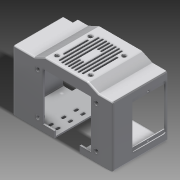
# Autodesk Inventor part: Simple3DPrintEnclosure02
Saved by Autodesk Inventor 2015 (Build 190159000, 159)
## iProperties
Created: 2015-09-24
Part Number: Simple3DPrintEnclosure02
Material: Aluminum 6061 Black Anodized
Document SubType Name: Modeling
Designer: -
Density: 2.71 g/cm^3
Appearance: Aluminum - Polished
Mass: 237.828 g
Surface Area: 585.089 cm^2
Volume: 87.7595 cm^3
Author: -
Autodesk Inventor part; units mm, degrees
ref_plane "YZ Plane" through (0, 0, 0) normal (1, 0, 0) x (0, 1, 0)
ref_plane "XZ Plane" through (0, 0, 0) normal (0, 1, 0) x (-1, 0, 0)
ref_plane "XY Plane" through (0, 0, 0) normal (0, 0, 1) x (1, 0, 0)
ref_plane "Work Plane1" through (-36.1295, 16.7619, 114.6398) normal (0, 0, 1) x (1, 0, 0)
sketch "Sketch3" plane through (-36.1295, 16.7619, 114.6398) normal (0, 0, 1) x (1, 0, 0)
  line L0 (55.17, 45.25) -> (-64.79, 45.25)
  line L1 (-64.79, 45.25) -> (-64.79, -34.1)
  line L2 (-64.79, -34.1) -> (55.17, -34.1)
  line L3 (55.17, -34.1) -> (55.17, 45.25)
  line L4 (28.95, 31.25) -> (28.95, -26.1)
  line L5 (-28.4, 31.25) -> (28.95, 31.25)
  line L6 (-28.4, -26.1) -> (-28.4, 31.25)
  line L7 (28.95, -26.1) -> (-28.4, -26.1)
  line L8 (28.95, 31.25) -> (-28.4, 31.25)
  line L9 (-28.4, 31.25) -> (-28.4, -26.1)
  line L10 (-28.4, -26.1) -> (28.95, -26.1)
  line L11 (28.95, -26.1) -> (28.95, 31.25)
  dimension "d196" = 14
  dimension "d197" = 26.22
  dimension "d198" = 8
  dimension "d199" = 36.39
  dimension "d200" = 57.35
  dimension "d201" = 57.35
  dimension "d249" = 119.96
  constraints: 24 end point, 4 parallel, 2 horizontal, 2 perpendicular
  measures "d196" distance between parallel lines of L0 L5
  measures "d197" distance between parallel lines of L3 L4
  measures "d198" distance between parallel lines of L2 L7
  measures "d199" distance between parallel lines of L1 L6
  measures "d200" distance between parallel lines of L5 L10
  measures "d201" distance between parallel lines of L6 L11
  measures "d249" distance between parallel lines of L3 L1
extrude "Extrusion3" add sketch "Sketch3" along normal blind 2
sketch "Sketch4" plane through (-36.1295, 16.7619, 114.6398) normal (0, 0, -1) x (-1, 0, 0)
  line L0 (-55.17, 45.25) -> (64.79, 45.25) projected
  line L1 (-55.17, -34.1) -> (-55.17, 45.25) projected
  line L2 (64.79, -34.1) -> (-55.17, -34.1) projected
  line L3 (64.79, 45.25) -> (64.79, -34.1) projected
  line L4 (-53.17, -32.1) -> (62.79, -32.1)
  line L5 (-23.5099, 42.25) -> (25.1599, 42.25)
  line L6 (64.79, -34.1) -> (-55.17, -34.1) construction
  line L7 (4.81, -34.1) -> (4.81, -47.8213) construction
  line L8 (29.4, 28.05) -> (-27.75, 28.05) construction
  line L9 (0.825, 28.05) -> (0.825, 13.0921) construction
  line L10 (-55.17, 45.25) -> (64.79, 45.25) projected
  line L11 (-24.7778, 41.9689) -> (-36.5722, 36.4691)
  line L12 (-37.8401, 36.188) -> (-53.17, 36.188)
  line L13 (26.4278, 41.9689) -> (38.2222, 36.4691)
  line L14 (39.4901, 36.188) -> (62.79, 36.188)
  line L15 (64.79, 45.25) -> (64.79, -34.1) projected
  arc A0 (-37.8401, 36.188) -> (-36.5722, 36.4691) centre (-37.8401, 39.188) ccw
  arc A1 (-23.5099, 42.25) -> (-24.7778, 41.9689) centre (-23.5099, 39.25) ccw
  arc A2 (26.4278, 41.9689) -> (25.1599, 42.25) centre (25.1599, 39.25) ccw
  arc A3 (38.2222, 36.4691) -> (39.4901, 36.188) centre (39.4901, 39.188) ccw
  line L16 (-55.17, 38.188) -> (-37.8401, 38.188)
  arc A4 (-37.8401, 38.188) -> (-37.4175, 38.2817) centre (-37.8401, 39.188) ccw
  line L17 (-37.4175, 38.2817) -> (-25.623, 43.7815)
  arc A5 (-23.5099, 44.25) -> (-25.623, 43.7815) centre (-23.5099, 39.25) ccw
  line L18 (-23.5099, 44.25) -> (25.1599, 44.25)
  arc A6 (27.273, 43.7815) -> (25.1599, 44.25) centre (25.1599, 39.25) ccw
  line L19 (27.273, 43.7815) -> (39.0675, 38.2817)
  arc A7 (39.0675, 38.2817) -> (39.4901, 38.188) centre (39.4901, 39.188) ccw
  line L20 (39.4901, 38.188) -> (64.79, 38.188)
  line L21 (62.79, -32.1) -> (62.79, 36.188)
  line L22 (-53.17, -32.1) -> (-53.17, 36.188)
  line L23 (-55.17, 38.188) -> (-55.17, -34.1)
  line L24 (64.79, -34.1) -> (64.79, 38.188)
  point P0 (-36.1295, -16.7619)
  point P1 (-24.175, 42.25)
  point P2 (25.825, 42.25)
  point P3 (-37.175, 36.188)
  point P4 (38.825, 36.188)
  point P5 (0.825, 42.25)
  dimension "d70" = 3
  dimension "d71" = 155
  dimension "d72" = 13
  dimension "d73" = 50
  dimension "d74" = 155
  dimension "d75" = 13
  dimension "d76" = 3
  dimension "d77" = 2
  dimension "d78" = 2
  dimension "d79" = 2
  dimension "d204" = 2
  dimension "d205" = 2
  dimension "d206" = 2
  dimension "d250" = 115.96
  dimension "d263" = 39.6301
  dimension "d264" = 31.6601
  dimension "d265" = 72.288
  constraints: 34 end point, 16 point on circle, 9 point on line, 8 centre point, 8 tangent, 3 equal radius, 3 horizontal, 3 midpoint, 2 collinear, 2 perpendicular, 2 vertical, 6 other
  measures "d70" distance between parallel lines of L5 L0
  measures "d71" angle of L11 L5
  measures "d72" horizontal distance of point (-37.175, 36.188) point (-24.175, 42.25)
  measures "d73" distance of point (-24.175, 42.25) point (25.825, 42.25)
  measures "d74" angle of L13 L5
  measures "d75" horizontal distance of point (25.825, 42.25) point (38.825, 36.188)
  measures "d76" radius of A0
  measures "d77" distance between parallel lines of L11 L17
  measures "d78" distance between parallel lines of L20 L14
  measures "d79" distance between parallel lines of L16 L12
  measures "d204" distance between parallel lines of L2 L4
  measures "d205" distance between parallel lines of L1 L22
  measures "d206" distance between parallel lines of L3 L21
  measures "d250" distance between parallel lines of L21 L22
  measures "d263" distance from line of L18.end L3
  measures "d264" distance from line of L1 L18.start
  measures "d265" distance between parallel lines of L2 L16
extrude "Extrusion4" add sketch "Sketch4" along normal blind 63 contours L16 A4 L17 A5 L18 A6 L19 A7 L20 L3 L2 L1
sketch "Sketch9" plane through (-36.1295, 16.7619, 114.6398) normal (0, 0, -1) x (-1, 0, 0)
  arc A0 (-23.5099, 44.25) -> (-25.623, 43.7815) centre (-23.5099, 39.25) ccw projected
  line L0 (-55.17, 45.25) -> (64.79, 45.25) projected
  line L1 (-55.17, 38.188) -> (-55.17, 45.25) projected
  line L2 (-55.17, 38.188) -> (-37.8401, 38.188) projected
  line L3 (-37.4175, 38.2817) -> (-25.623, 43.7815) projected
  arc A1 (27.273, 43.7815) -> (25.1599, 44.25) centre (25.1599, 39.25) ccw projected
  line L4 (27.273, 43.7815) -> (39.0675, 38.2817) projected
  line L5 (39.4901, 38.188) -> (64.79, 38.188) projected
  line L6 (64.79, 45.25) -> (64.79, 38.188) projected
  line L7 (-55.17, 45.25) -> (64.79, 45.25) projected
  line L8 (-55.17, 38.188) -> (-55.17, 45.25) projected
  line L9 (-55.17, 38.188) -> (-37.8401, 38.188) projected
  line L10 (-37.4175, 38.2817) -> (-25.623, 43.7815) projected
  arc A2 (-23.5099, 44.25) -> (-25.623, 43.7815) centre (-23.5099, 39.25) ccw projected
  line L11 (39.4901, 38.188) -> (64.79, 38.188) projected
  line L12 (64.79, 45.25) -> (64.79, 38.188) projected
  arc A3 (27.273, 43.7815) -> (25.1599, 44.25) centre (25.1599, 39.25) ccw projected
  line L13 (27.273, 43.7815) -> (39.0675, 38.2817) projected
  arc A4 (-37.8401, 38.188) -> (-37.4175, 38.2817) centre (-37.8401, 39.188) ccw projected
  line L14 (-23.5099, 44.25) -> (25.1599, 44.25) projected
  arc A5 (39.0675, 38.2817) -> (39.4901, 38.188) centre (39.4901, 39.188) ccw projected
  arc A6 (-37.8401, 38.188) -> (-37.4175, 38.2817) centre (-37.8401, 39.188) ccw projected
  line L15 (-23.5099, 44.25) -> (25.1599, 44.25) projected
  arc A7 (39.0675, 38.2817) -> (39.4901, 38.188) centre (39.4901, 39.188) ccw projected
  point P0 (-36.1295, -16.7619)
extrude "Extrusion9" cut sketch "Sketch9" against normal blind 6
fillet "Fillet16" radius 2 12 edges at (-100.9195, 54.9499, 84.1398) (19.0405, 54.9499, 84.1398) (19.0405, -17.3381, 84.1398) (-100.9195, -17.3381, 84.1398) (-88.2695, 54.9499, 116.6398) (-100.9195, 18.8059, 116.6398) (19.0405, 18.8059, 116.6398) (10.3756, 54.9499, 116.6398) (-11.5374, 60.8934, 116.6398) (-62.3716, 60.8934, 116.6398) (-69.2997, 57.7936, 116.6398) (-4.6093, 57.7936, 116.6398)
chamfer "Chamfer1" [suppressed]
chamfer "Chamfer2" [suppressed]
chamfer "Chamfer5" [suppressed]
fillet "Fillet5" [suppressed]
fillet "Fillet6" [suppressed]
fillet "Fillet14" [suppressed]
sketch "Sketch7" plane through (19.0405, -15.3381, 51.6398) normal (1, 0, 0) x (0, 0, -1)
  line L0 (-40, 62) -> (-4, 62)
  line L1 (-2, 60) -> (-2, 9)
  line L2 (-4, 7) -> (-40, 7)
  line L3 (-42, 9) -> (-42, 60)
  arc A0 (-40, 62) -> (-42, 60) centre (-40, 60) ccw
  arc A1 (-2, 60) -> (-4, 62) centre (-4, 60) ccw
  arc A2 (-4, 7) -> (-2, 9) centre (-4, 9) ccw
  arc A3 (-42, 9) -> (-40, 7) centre (-40, 9) ccw
  line L4 (0, 68.288) -> (0, 0) projected
  line L5 (-64, -2) -> (0, -2) projected
  point P0 (51.6398, 15.3381)
  point P1 (0, 69.288)
  point P2 (-64.7639, -2)
  point P3 (-63.5279, -2)
  dimension "d46" = 2
  dimension "d65" = 40
  dimension "d66" = 55
  dimension "d240" = 2
  dimension "d241" = 9
  constraints: 8 end point, 8 point on circle, 8 tangent, 4 centre point, 3 equal radius, 2 parallel, 1 horizontal, 1 perpendicular
  measures "d46" radius of A0
  measures "d65" distance between parallel lines of L3 L1
  measures "d66" distance between parallel lines of L2 L0
  measures "d240" distance between parallel lines of L1 L4
  measures "d241" distance between parallel lines of L5 L2
extrude "Extrusion7" cut sketch "Sketch7" against normal blind 1
lip "Lip1" kind groove height 1 width 1 edges at (-40.9395, -15.3381, 51.6398) (-98.9195, 18.8059, 51.6398) (-87.2695, 52.9499, 51.6398) (-74.9703, 53.021, 51.6398) (-68.4545, 55.9809, 51.6398) (-61.9387, 58.9408, 51.6398) (-36.9545, 59.0119, 51.6398) (-11.9703, 58.9408, 51.6398) (-5.4545, 55.9809, 51.6398) (1.0613, 53.021, 51.6398) (9.3756, 52.9499, 51.6398) (17.0405, 18.8059, 51.6398) guide face at (-60.2662, -16.0047, 51.6398)
sketch "Sketch16" plane through (18.0405, -15.3381, 51.6398) normal (1, 0, 0) x (0, 0, -1)
  line L0 (-2, 60) -> (-2, 9) projected
  line L1 (-42, 58) -> (-2, 58)
  line L2 (-2, 58) -> (-2, 11)
  line L3 (-2, 11) -> (-42, 11)
  line L4 (-42, 11) -> (-42, 58)
  line L5 (-40, 62) -> (-4, 62) projected
  line L6 (-4, 7) -> (-40, 7) projected
  line L7 (-42, 9) -> (-42, 60) projected
  circle A0 centre (-22, 9) radius 1
  line L8 (-22, 11) -> (-22, 7) construction
  line L9 (-4, 7) -> (-40, 7) construction
  circle A1 centre (-22, 60) radius 1
  line L10 (-22, 58) -> (-22, 62) construction
  point P0 (51.6398, 15.3381)
  dimension "d243" = 4
  dimension "d244" = 4
  dimension "d247" = 2
  dimension "d248" = 2
  constraints: 12 end point, 7 midpoint, 2 centre point, 2 coincident, 2 parallel, 1 collinear, 1 horizontal, 1 perpendicular, 1 point on line
  measures "d243" distance between parallel lines of L5 L1
  measures "d244" distance between parallel lines of L6 L3
  measures "d247" diameter of A0
  measures "d248" diameter of A1
extrude "Extrusion15" cut sketch "Sketch16" against normal blind 10
sketch "Sketch8" plane through (-36.1295, 16.7619, 116.6398) normal (0, 0, 1) x (1, 0, 0)
  circle A0 centre (-34.95, 27.44) radius 1.5
  circle A1 centre (-34.95, -22.29) radius 1.5
  line L0 (0, 0) -> (0, 75.8555) construction
  circle A2 centre (34.95, 27.44) radius 1.5
  circle A3 centre (34.95, -22.29) radius 1.5
  line L1 (0, 0) -> (67.5955, 0) construction
  line L2 (-28.4, 31.25) -> (28.95, 31.25) projected
  line L3 (28.95, 31.25) -> (28.95, -26.1) projected
  line L4 (28.95, -26.1) -> (-28.4, -26.1) projected
  point P0 (0, 28.05)
  dimension "d55" = 3
  dimension "d58" = 3
  dimension "d259" = 3.81
  dimension "d260" = 6
  dimension "d261" = 6
  dimension "d262" = 3.81
  constraints: 4 centre point, 4 end point, 2 point on line, 2 symmetric about line, 1 horizontal, 1 vertical, 3 other
  measures "d55" diameter of A0
  measures "d58" diameter of A1
  measures "d259" distance from line of A2.centre L2
  measures "d260" distance from line of A2.centre L3
  measures "d261" distance from line of L3 A3.centre
  measures "d262" distance from line of L4 A3.centre
extrude "Extrusion8" cut sketch "Sketch8" against normal blind 6
chamfer "Chamfer4" distance 1.2 angle 45 4 edges at (-72.5795, 44.2019, 116.6398) (-72.5795, -5.5281, 116.6398) (-2.6795, 44.2019, 116.6398) (-2.6795, -5.5281, 116.6398)
fillet "Fillet11" radius 1 4 edges at (-3.8795, -5.5281, 116.6398) (-3.8795, 44.2019, 116.6398) (-73.7795, 44.2019, 116.6398) (-73.7795, -5.5281, 116.6398)
fillet "Fillet12" radius 2 8 edges at (-98.9195, -15.3381, 83.6398) (-99.9195, -16.3381, 52.1398) (17.0405, -15.3381, 83.6398) (18.0405, -16.3381, 52.1398) (17.0405, 52.9499, 83.6398) (18.0405, 53.9499, 52.1398) (-98.9195, 52.9499, 83.6398) (-99.9195, 53.9499, 52.1398)
sketch "Sketch10" plane through (-61.2894, 61.0119, 51.6398) normal (0, 1, 0) x (1, 0, 0)
  line L0 (49.1988, -64.7639) -> (-0.8012, -64.7639) construction
  line L1 (-0.8012, -64.7639) -> (-0.8012, -14.7639) construction
  line L2 (-0.8012, -14.7639) -> (49.1988, -14.7639) construction
  line L3 (49.1988, -14.7639) -> (49.1988, -64.7639) construction
  line L4 (48.6698, -64) -> (48.6698, 0) construction
  line L5 (0, 0) -> (48.6698, 0) construction
  line L6 (0, -64) -> (0, 0) construction
  circle A0 centre (4.1988, -15.7639) radius 1.75
  line L7 (48.6698, 0) -> (0, 0) construction
  line L8 (24.3349, 0) -> (24.3349, 10.9625) construction
  circle A1 centre (44.471, -15.7639) radius 1.75
  circle A2 centre (4.1988, -55.7639) radius 1.75
  circle A3 centre (44.471, -55.7639) radius 1.75
  line L9 (42.221, -50.7639) -> (42.221, -50.7639)
  line L10 (43.221, -49.7639) -> (43.221, -21.7639)
  line L11 (42.221, -20.7639) -> (42.221, -20.7639)
  line L12 (41.221, -21.7639) -> (41.221, -49.7639)
  line L13 (39.2176, -35.7639) -> (24.1918, -35.7639) construction
  line L14 (44.471, -55.7639) -> (44.471, -15.7639) construction
  arc A4 (41.221, -49.7639) -> (42.221, -50.7639) centre (42.221, -49.7639) ccw
  arc A5 (42.221, -50.7639) -> (43.221, -49.7639) centre (42.221, -49.7639) ccw
  arc A6 (43.221, -21.7639) -> (42.221, -20.7639) centre (42.221, -21.7639) ccw
  arc A7 (42.221, -20.7639) -> (41.221, -21.7639) centre (42.221, -21.7639) ccw
  line L15 (38.221, -59.7639) -> (38.221, -59.7639)
  line L16 (39.221, -58.7639) -> (39.221, -12.7639)
  line L17 (38.221, -11.7639) -> (38.221, -11.7639)
  line L18 (37.221, -12.7639) -> (37.221, -58.7639)
  arc A8 (37.221, -58.7639) -> (38.221, -59.7639) centre (38.221, -58.7639) ccw
  arc A9 (38.221, -59.7639) -> (39.221, -58.7639) centre (38.221, -58.7639) ccw
  arc A10 (39.221, -12.7639) -> (38.221, -11.7639) centre (38.221, -12.7639) ccw
  arc A11 (38.221, -11.7639) -> (37.221, -12.7639) centre (38.221, -12.7639) ccw
  line L19 (34.221, -60.7639) -> (34.221, -60.7639)
  line L20 (35.221, -59.7639) -> (35.221, -11.7639)
  line L21 (34.221, -10.7639) -> (34.221, -10.7639)
  line L22 (33.221, -11.7639) -> (33.221, -59.7639)
  arc A12 (33.221, -59.7639) -> (34.221, -60.7639) centre (34.221, -59.7639) ccw
  arc A13 (34.221, -60.7639) -> (35.221, -59.7639) centre (34.221, -59.7639) ccw
  arc A14 (35.221, -11.7639) -> (34.221, -10.7639) centre (34.221, -11.7639) ccw
  arc A15 (34.221, -10.7639) -> (33.221, -11.7639) centre (34.221, -11.7639) ccw
  line L23 (26.221, -10.7639) -> (26.221, -10.7639)
  line L24 (27.221, -11.7639) -> (27.221, -24.7639)
  line L25 (26.221, -25.7639) -> (26.221, -25.7639)
  line L26 (25.221, -24.7639) -> (25.221, -11.7639)
  arc A16 (26.221, -10.7639) -> (25.221, -11.7639) centre (26.221, -11.7639) ccw
  arc A17 (27.221, -11.7639) -> (26.221, -10.7639) centre (26.221, -11.7639) ccw
  arc A18 (26.221, -25.7639) -> (27.221, -24.7639) centre (26.221, -24.7639) ccw
  arc A19 (25.221, -24.7639) -> (26.221, -25.7639) centre (26.221, -24.7639) ccw
  line L27 (49.471, -14.7639) -> (-0.529, -14.7639) construction
  line L28 (22.4488, -10.7639) -> (22.4488, -10.7639)
  line L29 (21.4488, -11.7639) -> (21.4488, -24.7639)
  line L30 (22.4488, -25.7639) -> (22.4488, -25.7639)
  line L31 (23.4488, -24.7639) -> (23.4488, -11.7639)
  arc A20 (23.4488, -11.7639) -> (22.4488, -10.7639) centre (22.4488, -11.7639) ccw
  arc A21 (22.4488, -10.7639) -> (21.4488, -11.7639) centre (22.4488, -11.7639) ccw
  arc A22 (21.4488, -24.7639) -> (22.4488, -25.7639) centre (22.4488, -24.7639) ccw
  arc A23 (22.4488, -25.7639) -> (23.4488, -24.7639) centre (22.4488, -24.7639) ccw
  line L32 (30.221, -60.7639) -> (30.221, -60.7639)
  line L33 (31.221, -59.7639) -> (31.221, -11.7639)
  line L34 (30.221, -10.7639) -> (30.221, -10.7639)
  line L35 (29.221, -11.7639) -> (29.221, -59.7639)
  arc A24 (29.221, -59.7639) -> (30.221, -60.7639) centre (30.221, -59.7639) ccw
  arc A25 (30.221, -60.7639) -> (31.221, -59.7639) centre (30.221, -59.7639) ccw
  arc A26 (31.221, -11.7639) -> (30.221, -10.7639) centre (30.221, -11.7639) ccw
  arc A27 (30.221, -10.7639) -> (29.221, -11.7639) centre (30.221, -11.7639) ccw
  line L36 (26.221, -45.7639) -> (26.221, -45.7639)
  line L37 (27.221, -46.7639) -> (27.221, -59.7639)
  line L38 (26.221, -60.7639) -> (26.221, -60.7639)
  line L39 (25.221, -59.7639) -> (25.221, -46.7639)
  arc A28 (26.221, -45.7639) -> (25.221, -46.7639) centre (26.221, -46.7639) ccw
  arc A29 (27.221, -46.7639) -> (26.221, -45.7639) centre (26.221, -46.7639) ccw
  arc A30 (26.221, -60.7639) -> (27.221, -59.7639) centre (26.221, -59.7639) ccw
  arc A31 (25.221, -59.7639) -> (26.221, -60.7639) centre (26.221, -59.7639) ccw
  arc A32 (22.4488, -45.7639) -> (21.4488, -46.7639) centre (22.4488, -46.7639) ccw
  line L40 (22.4488, -45.7639) -> (22.4488, -45.7639)
  arc A33 (23.4488, -46.7639) -> (22.4488, -45.7639) centre (22.4488, -46.7639) ccw
  line L41 (21.4488, -46.7639) -> (21.4488, -59.7639)
  line L42 (23.4488, -59.7639) -> (23.4488, -46.7639)
  arc A34 (22.4488, -60.7639) -> (23.4488, -59.7639) centre (22.4488, -59.7639) ccw
  line L43 (22.4488, -60.7639) -> (22.4488, -60.7639)
  arc A35 (21.4488, -59.7639) -> (22.4488, -60.7639) centre (22.4488, -59.7639) ccw
  line L44 (18.721, -60.7639) -> (18.721, -60.7639)
  line L45 (19.721, -59.7639) -> (19.721, -11.7639)
  line L46 (18.721, -10.7639) -> (18.721, -10.7639)
  line L47 (17.721, -11.7639) -> (17.721, -59.7639)
  arc A36 (17.721, -59.7639) -> (18.721, -60.7639) centre (18.721, -59.7639) ccw
  arc A37 (18.721, -60.7639) -> (19.721, -59.7639) centre (18.721, -59.7639) ccw
  arc A38 (19.721, -11.7639) -> (18.721, -10.7639) centre (18.721, -11.7639) ccw
  arc A39 (18.721, -10.7639) -> (17.721, -11.7639) centre (18.721, -11.7639) ccw
  line L48 (14.721, -60.7639) -> (14.721, -60.7639)
  line L49 (15.721, -59.7639) -> (15.721, -11.7639)
  line L50 (14.721, -10.7639) -> (14.721, -10.7639)
  line L51 (13.721, -11.7639) -> (13.721, -59.7639)
  arc A40 (13.721, -59.7639) -> (14.721, -60.7639) centre (14.721, -59.7639) ccw
  arc A41 (14.721, -60.7639) -> (15.721, -59.7639) centre (14.721, -59.7639) ccw
  arc A42 (15.721, -11.7639) -> (14.721, -10.7639) centre (14.721, -11.7639) ccw
  arc A43 (14.721, -10.7639) -> (13.721, -11.7639) centre (14.721, -11.7639) ccw
  line L52 (10.721, -59.7639) -> (10.721, -59.7639)
  line L53 (11.721, -58.7639) -> (11.721, -12.7639)
  line L54 (10.721, -11.7639) -> (10.721, -11.7639)
  line L55 (9.721, -12.7639) -> (9.721, -58.7639)
  arc A44 (9.721, -58.7639) -> (10.721, -59.7639) centre (10.721, -58.7639) ccw
  arc A45 (10.721, -59.7639) -> (11.721, -58.7639) centre (10.721, -58.7639) ccw
  arc A46 (11.721, -12.7639) -> (10.721, -11.7639) centre (10.721, -12.7639) ccw
  arc A47 (10.721, -11.7639) -> (9.721, -12.7639) centre (10.721, -12.7639) ccw
  line L56 (6.721, -50.7639) -> (6.721, -50.7639)
  line L57 (7.721, -49.7639) -> (7.721, -21.7639)
  line L58 (6.721, -20.7639) -> (6.721, -20.7639)
  line L59 (5.721, -21.7639) -> (5.721, -49.7639)
  arc A48 (5.721, -49.7639) -> (6.721, -50.7639) centre (6.721, -49.7639) ccw
  arc A49 (6.721, -50.7639) -> (7.721, -49.7639) centre (6.721, -49.7639) ccw
  arc A50 (7.721, -21.7639) -> (6.721, -20.7639) centre (6.721, -21.7639) ccw
  arc A51 (6.721, -20.7639) -> (5.721, -21.7639) centre (6.721, -21.7639) ccw
  line L60 (48.6698, -64) -> (0, -64)
  point P0 (61.2894, 51.6398)
  point P1 (24.1988, -64.7639)
  point P2 (49.061, -66.2512)
  point P3 (41.221, -35.7639)
  point P4 (44.471, -35.7639)
  point P5 (39.221, -11.7639)
  point P6 (39.221, -59.7639)
  point P7 (37.221, -11.7639)
  point P8 (37.221, -35.7639)
  point P9 (35.221, -10.7639)
  point P10 (35.221, -60.7639)
  point P11 (33.221, -10.7639)
  point P12 (33.221, -35.7639)
  point P13 (27.221, -25.7639)
  point P14 (27.221, -10.7639)
  point P15 (25.221, -25.7639)
  point P16 (21.4488, -25.7639)
  point P17 (21.4488, -10.7639)
  point P18 (23.4488, -25.7639)
  point P19 (31.221, -10.7639)
  point P20 (31.221, -60.7639)
  point P21 (29.221, -10.7639)
  point P22 (29.221, -35.7639)
  point P23 (27.221, -60.7639)
  point P24 (27.221, -45.7639)
  point P25 (25.221, -60.7639)
  point P26 (21.4488, -45.7639)
  point P27 (23.4488, -60.7639)
  point P28 (21.4488, -60.7639)
  point P29 (19.721, -10.7639)
  point P30 (19.721, -60.7639)
  point P31 (17.721, -10.7639)
  point P32 (17.721, -35.7639)
  point P33 (15.721, -10.7639)
  point P34 (15.721, -60.7639)
  point P35 (13.721, -10.7639)
  point P36 (13.721, -35.7639)
  point P37 (11.7176, -35.7639)
  point P38 (11.721, -11.7639)
  point P39 (11.721, -59.7639)
  point P40 (9.721, -11.7639)
  point P41 (9.721, -35.7639)
  point P42 (5.721, -35.7639)
  dimension "d87" = 50
  dimension "d88" = 50
  dimension "d108" = 3.5
  dimension "d109" = 5
  dimension "d112" = 40
  dimension "d117" = 40
  dimension "d118" = 40.2722
  dimension "d119" = 9
  dimension "d121" = 30
  dimension "d123" = 2
  dimension "d124" = 1
  dimension "d125" = 2.5
  dimension "d131" = 2
  dimension "d132" = 48
  dimension "d133" = 2
  dimension "d134" = 1
  dimension "d135" = 2
  dimension "d136" = 50
  dimension "d137" = 2
  dimension "d138" = 1
  dimension "d147" = 2
  dimension "d148" = 15
  dimension "d151" = 1
  dimension "d152" = 2
  dimension "d153" = 50
  dimension "d154" = 2
  dimension "d155" = 1
  dimension "d156" = 2
  dimension "d157" = 1
  dimension "d160" = 35
  dimension "d167" = 15.5
  dimension "d172" = 9.5
  dimension "d175" = 27.5
  dimension "d180" = 2
  dimension "d183" = 35.5
  dimension "d188" = 2
  constraints: 122 end point, 96 point on circle, 65 point on line, 52 centre point, 40 tangent, 18 symmetric about line, 15 equal radius, 12 parallel, 9 horizontal, 7 midpoint, 7 perpendicular, 3 vertical, 124 other
  measures "d87" distance of L1.end L2.end
  measures "d88" distance of L0.end L1.end
  measures "d108" diameter of A0
  measures "d109" distance from line of A0.centre L1
  measures "d112" distance of A0.centre A2.centre
  measures "d117" distance of L14.start L14.end
  measures "d118" distance of L14.end A0.centre
  measures "d119" distance from line of A2.centre L0
  measures "d121" distance between parallel lines of L11 L9
  measures "d123" distance between parallel lines of L10 L12
  measures "d124" radius of A4
  measures "d125" diameter of L10 L14
  measures "d131" distance of point (37.221, -11.764) point (39.221, -11.764)
  measures "d132" distance of point (39.221, -11.764) point (39.221, -59.764)
  measures "d133" distance between parallel lines of L12 L16
  measures "d134" radius of A8
  measures "d135" distance of point (33.221, -10.764) point (35.221, -10.764)
  measures "d136" distance of point (35.221, -10.764) point (35.221, -60.764)
  measures "d137" distance between parallel lines of L20 L18
  measures "d138" radius of A12
  measures "d147" distance of point (27.221, -25.764) point (25.221, -25.764)
  measures "d148" distance of point (27.221, -10.764) point (27.221, -25.764)
  measures "d151" radius of A16
  measures "d152" distance of point (29.221, -10.764) point (31.221, -10.764)
  measures "d153" distance of point (31.221, -10.764) point (31.221, -60.764)
  measures "d154" distance between parallel lines of L22 L33
  measures "d155" radius of A24
  measures "d156" distance between parallel lines of L24 L35
  measures "d157" vertical distance of point (29.221, -10.764) A17.centre
  measures "d160" distance of L24.start L37.start
  measures "d167" distance of point (29.221, -35.764) point (13.721, -35.764)
  measures "d172" distance between parallel lines of L35 L45
  measures "d175" distance of point (37.221, -11.764) point (9.721, -11.764)
  measures "d180" distance between parallel lines of L51 L53
  measures "d183" distance of L11.start L58.start
  measures "d188" distance between parallel lines of L57 L55
extrude "Extrusion10" cut sketch "Sketch10" against normal blind 10
sketch "Sketch11" plane through (-97.9195, -17.3381, 51.6398) normal (0, -1, 0) x (1, 0, 0)
  line L0 (62.065, 68) -> (62.065, 29.2393) construction
  line L1 (46.965, 65) -> (77.165, 65)
  line L2 (77.165, 65) -> (77.165, 20.9)
  line L3 (77.165, 20.9) -> (46.965, 20.9)
  line L4 (46.965, 20.9) -> (46.965, 65)
  line L5 (90.74, 65) -> (33.39, 65) projected
  point P0 (97.9195, -51.6398)
  point P1 (62.065, 65)
  point P2 (62.065, 65)
  dimension "d104" = 30.2
  dimension "d266" = 44.1
  constraints: 10 end point, 2 midpoint, 2 parallel, 2 point on line, 1 collinear, 1 horizontal, 1 perpendicular, 1 vertical
  measures "d104" distance of L1.start L1.end
  measures "d266" distance between parallel lines of L3 L1
extrude "Extrusion11" cut sketch "Sketch11" against normal blind 10
sketch "Sketch13" plane through (-36.1295, 16.7619, 114.6398) normal (0, 0, -1) x (-1, 0, 0)
  line L0 (40.7978, -31.225) -> (64.4775, -31.225) projected
  line L1 (43.8489, 33.1934) -> (43.8489, -32.2839)
  point P0 (-36.1295, -16.7619)
  point P1 (64.4775, -31.1)
  point P2 (40.7978, -31.1)
  constraints: 2 end point, 1 perpendicular
extrude "Extrusion12" [suppressed]
fillet "Fillet13" [suppressed]
chamfer "Chamfer6" distance 1 angle 45 4 edges at (-18.5684, 61.0119, 67.4038) (-18.5684, 61.0119, 107.4038) (-58.8406, 61.0119, 107.4038) (-58.8406, 61.0119, 67.4038)
sketch "Sketch14" plane through (-36.1295, 16.7619, 116.6398) normal (0, 0, 1) x (1, 0, 0)
  line L0 (41.95, 30.188) -> (43.17, 30.188)
  line L1 (47.17, 26.188) -> (47.17, -21.1)
  line L2 (43.17, -25.1) -> (41.95, -25.1)
  line L3 (37.95, -21.1) -> (37.95, 26.188)
  line L4 (28.95, 31.25) -> (28.95, -26.1) projected
  line L5 (52.3481, 39.188) -> (38.2835, 39.188) projected
  line L6 (15.375, -34.1) -> (-14.825, -34.1) projected
  line L7 (55.17, -32.1) -> (55.17, 37.188) projected
  arc A0 (37.95, -21.1) -> (41.95, -25.1) centre (41.95, -21.1) ccw
  arc A1 (43.17, -25.1) -> (47.17, -21.1) centre (43.17, -21.1) ccw
  arc A2 (47.17, 26.188) -> (43.17, 30.188) centre (43.17, 26.188) ccw
  arc A3 (41.95, 30.188) -> (37.95, 26.188) centre (41.95, 26.188) ccw
  point P0 (36.1295, -16.7619)
  point P1 (52.3547, 39.188)
  point P2 (53.17, -34.1)
  point P3 (42.56, -17.1468)
  point P4 (42.56, 22.2348)
  dimension "d220" = 9
  dimension "d221" = 9
  dimension "d222" = 9
  dimension "d223" = 8
  dimension "d224" = 4
  constraints: 12 point on circle, 8 end point, 8 tangent, 4 centre point, 3 equal radius, 2 parallel, 1 horizontal, 1 perpendicular
  measures "d220" distance between parallel lines of L4 L3
  measures "d221" distance between parallel lines of L5 L0
  measures "d222" distance between parallel lines of L6 L2
  measures "d223" distance between parallel lines of L7 L1
  measures "d224" radius of A0
extrude "Extrusion13" [suppressed]
fillet "Fillet15" [suppressed]
sketch "Sketch15" plane through (-98.9195, -17.3381, 51.6398) normal (0, -1, 0) x (1, 0, 0)
  line L0 (84.165, 56.8944) -> (85.165, 56.8944)
  line L1 (86.165, 55.8944) -> (86.165, 53)
  line L2 (85.165, 52) -> (84.165, 52)
  line L3 (83.165, 53) -> (83.165, 55.8944)
  line L4 (78.165, 65) -> (78.165, 20.9) projected
  line L5 (78.165, 66.8944) -> (47.965, 66.8944) projected
  line L6 (115.96, 0) -> (0, 0) projected
  arc A0 (84.165, 56.8944) -> (83.165, 55.8944) centre (84.165, 55.8944) ccw
  arc A1 (86.165, 55.8944) -> (85.165, 56.8944) centre (85.165, 55.8944) ccw
  arc A2 (83.165, 53) -> (84.165, 52) centre (84.165, 53) ccw
  arc A3 (85.165, 52) -> (86.165, 53) centre (85.165, 53) ccw
  line L7 (41.965, 56.8944) -> (40.965, 56.8944)
  line L8 (39.965, 55.8944) -> (39.965, 53)
  line L9 (40.965, 52) -> (41.965, 52)
  line L10 (42.965, 53) -> (42.965, 55.8944)
  line L11 (1.2361, 66.8944) -> (47.965, 66.8944) projected
  line L12 (47.965, 20.9) -> (47.965, 65) projected
  arc A4 (40.965, 56.8944) -> (39.965, 55.8944) centre (40.965, 55.8944) ccw
  arc A5 (42.965, 55.8944) -> (41.965, 56.8944) centre (41.965, 55.8944) ccw
  arc A6 (41.965, 52) -> (42.965, 53) centre (41.965, 53) ccw
  arc A7 (39.965, 53) -> (40.965, 52) centre (40.965, 53) ccw
  line L13 (84.165, 41.8944) -> (85.165, 41.8944)
  line L14 (86.165, 40.8944) -> (86.165, 38)
  line L15 (85.165, 37) -> (84.165, 37)
  line L16 (83.165, 38) -> (83.165, 40.8944)
  arc A8 (84.165, 41.8944) -> (83.165, 40.8944) centre (84.165, 40.8944) ccw
  arc A9 (86.165, 40.8944) -> (85.165, 41.8944) centre (85.165, 40.8944) ccw
  arc A10 (83.165, 38) -> (84.165, 37) centre (84.165, 38) ccw
  arc A11 (85.165, 37) -> (86.165, 38) centre (85.165, 38) ccw
  line L17 (41.965, 41.8944) -> (40.965, 41.8944)
  line L18 (39.965, 40.8944) -> (39.965, 38)
  line L19 (40.965, 37) -> (41.965, 37)
  line L20 (42.965, 38) -> (42.965, 40.8944)
  arc A12 (40.965, 41.8944) -> (39.965, 40.8944) centre (40.965, 40.8944) ccw
  arc A13 (42.965, 40.8944) -> (41.965, 41.8944) centre (41.965, 40.8944) ccw
  arc A14 (41.965, 37) -> (42.965, 38) centre (41.965, 38) ccw
  arc A15 (39.965, 38) -> (40.965, 37) centre (40.965, 38) ccw
  line L21 (84.165, 26.8944) -> (85.165, 26.8944)
  line L22 (86.165, 25.8944) -> (86.165, 23)
  line L23 (85.165, 22) -> (84.165, 22)
  line L24 (83.165, 23) -> (83.165, 25.8944)
  arc A16 (84.165, 26.8944) -> (83.165, 25.8944) centre (84.165, 25.8944) ccw
  arc A17 (86.165, 25.8944) -> (85.165, 26.8944) centre (85.165, 25.8944) ccw
  arc A18 (83.165, 23) -> (84.165, 22) centre (84.165, 23) ccw
  arc A19 (85.165, 22) -> (86.165, 23) centre (85.165, 23) ccw
  line L25 (41.965, 26.8944) -> (40.965, 26.8944)
  line L26 (39.965, 25.8944) -> (39.965, 23)
  line L27 (40.965, 22) -> (41.965, 22)
  line L28 (42.965, 23) -> (42.965, 25.8944)
  arc A20 (40.965, 26.8944) -> (39.965, 25.8944) centre (40.965, 25.8944) ccw
  arc A21 (42.965, 25.8944) -> (41.965, 26.8944) centre (41.965, 25.8944) ccw
  arc A22 (41.965, 22) -> (42.965, 23) centre (41.965, 23) ccw
  arc A23 (39.965, 23) -> (40.965, 22) centre (40.965, 23) ccw
  line L29 (92.165, 56.8944) -> (93.165, 56.8944)
  line L30 (94.165, 55.8944) -> (94.165, 53)
  line L31 (93.165, 52) -> (92.165, 52)
  line L32 (91.165, 53) -> (91.165, 55.8944)
  arc A24 (92.165, 56.8944) -> (91.165, 55.8944) centre (92.165, 55.8944) ccw
  arc A25 (94.165, 55.8944) -> (93.165, 56.8944) centre (93.165, 55.8944) ccw
  arc A26 (91.165, 53) -> (92.165, 52) centre (92.165, 53) ccw
  arc A27 (93.165, 52) -> (94.165, 53) centre (93.165, 53) ccw
  line L33 (93.165, 37) -> (92.165, 37)
  arc A28 (93.165, 37) -> (94.165, 38) centre (93.165, 38) ccw
  arc A29 (91.165, 38) -> (92.165, 37) centre (92.165, 38) ccw
  line L34 (94.165, 40.8944) -> (94.165, 38)
  line L35 (91.165, 38) -> (91.165, 40.8944)
  arc A30 (94.165, 40.8944) -> (93.165, 41.8944) centre (93.165, 40.8944) ccw
  line L36 (92.165, 41.8944) -> (93.165, 41.8944)
  arc A31 (92.165, 41.8944) -> (91.165, 40.8944) centre (92.165, 40.8944) ccw
  line L37 (93.165, 22) -> (92.165, 22)
  arc A32 (93.165, 22) -> (94.165, 23) centre (93.165, 23) ccw
  arc A33 (91.165, 23) -> (92.165, 22) centre (92.165, 23) ccw
  line L38 (94.165, 25.8944) -> (94.165, 23)
  line L39 (91.165, 23) -> (91.165, 25.8944)
  arc A34 (94.165, 25.8944) -> (93.165, 26.8944) centre (93.165, 25.8944) ccw
  line L40 (92.165, 26.8944) -> (93.165, 26.8944)
  arc A35 (92.165, 26.8944) -> (91.165, 25.8944) centre (92.165, 25.8944) ccw
  line L41 (33.965, 56.8944) -> (32.965, 56.8944)
  line L42 (31.965, 55.8944) -> (31.965, 53)
  line L43 (32.965, 52) -> (33.965, 52)
  line L44 (34.965, 53) -> (34.965, 55.8944)
  arc A36 (32.965, 56.8944) -> (31.965, 55.8944) centre (32.965, 55.8944) ccw
  arc A37 (34.965, 55.8944) -> (33.965, 56.8944) centre (33.965, 55.8944) ccw
  arc A38 (33.965, 52) -> (34.965, 53) centre (33.965, 53) ccw
  arc A39 (31.965, 53) -> (32.965, 52) centre (32.965, 53) ccw
  arc A40 (34.965, 40.8944) -> (33.965, 41.8944) centre (33.965, 40.8944) ccw
  arc A41 (33.965, 37) -> (34.965, 38) centre (33.965, 38) ccw
  line L45 (32.965, 37) -> (33.965, 37)
  line L46 (33.965, 41.8944) -> (32.965, 41.8944)
  arc A42 (31.965, 38) -> (32.965, 37) centre (32.965, 38) ccw
  line L47 (31.965, 40.8944) -> (31.965, 38)
  arc A43 (32.965, 41.8944) -> (31.965, 40.8944) centre (32.965, 40.8944) ccw
  line L48 (34.965, 38) -> (34.965, 40.8944)
  arc A44 (34.965, 25.8944) -> (33.965, 26.8944) centre (33.965, 25.8944) ccw
  arc A45 (33.965, 22) -> (34.965, 23) centre (33.965, 23) ccw
  line L49 (32.965, 22) -> (33.965, 22)
  line L50 (33.965, 26.8944) -> (32.965, 26.8944)
  arc A46 (31.965, 23) -> (32.965, 22) centre (32.965, 23) ccw
  line L51 (31.965, 25.8944) -> (31.965, 23)
  arc A47 (32.965, 26.8944) -> (31.965, 25.8944) centre (32.965, 25.8944) ccw
  line L52 (34.965, 23) -> (34.965, 25.8944)
  point P0 (98.9195, -51.6398)
  point P1 (78.165, 63.5279)
  point P2 (78.165, 66.8944)
  point P3 (113.4879, 67.7889)
  point P4 (2.4721, 67.7889)
  point P5 (47.965, 63.5279)
  point P6 (78.165, 64)
  point P7 (47.965, 64)
  point P8 (78.165, 66)
  point P9 (47.965, 66)
  dimension "d228" = 3
  dimension "d229" = 5
  dimension "d230" = 10
  dimension "d231" = 52
  dimension "d232" = 1
  dimension "d233" = 10
  dimension "d234" = 5
  dimension "d235" = 3
  dimension "d236" = 52
  dimension "d237" = 1
  dimension "d269" = 15
  dimension "d276" = 8
  dimension "d283" = 8
  constraints: 96 end point, 96 point on circle, 48 centre point, 16 tangent, 6 equal radius, 4 horizontal, 4 parallel, 3 collinear, 2 perpendicular, 1 vertical, 199 other
  measures "d228" distance between parallel lines of L3 L1
  measures "d229" distance between parallel lines of L4 L3
  measures "d231" distance between parallel lines of L6 L2
  measures "d232" radius of A0
  measures "d234" distance between parallel lines of L10 L12
  measures "d235" distance between parallel lines of L8 L10
  measures "d236" distance between parallel lines of L6 L9
  measures "d237" radius of A4
  measures "d269" distance of L2.start L15.start
  measures "d276" distance of L0.start L29.start
  measures "d283" distance of L8.start L42.start
extrude "Extrusion14" cut sketch "Sketch15" against normal blind 5
sketch "Sketch17" plane through (-61.2894, 62.0119, 51.6398) normal (0, 1, 0) x (1, 0, 0)
  circle A0 centre (11.9349, -65.333) radius 1.5
  circle A1 centre (38.9349, -65.333) radius 1.5
  line L0 (0, -68) -> (48.6698, -68) projected
  line L1 (40.5349, -63) -> (40.5349, -66) projected
  line L2 (11.9349, -65.333) -> (38.9349, -65.333)
  line L3 (-3.2401, -66) -> (54.1099, -66) projected
  line L4 (25.4349, -66) -> (25.4349, -36.2927)
  line L5 (25.4349, -66) -> (55.1422, -66) construction
  point P0 (61.2894, 51.6398)
  point P1 (25.4349, -65.333)
  point P2 (54.1099, -66)
  dimension "d288" = 3
  dimension "d289" = 3
  dimension "d290" = 27
  dimension "d291" = 2.667
  dimension "d292" = 2.667
  dimension "d293" = 90
  constraints: 6 end point, 2 centre point, 1 horizontal, 1 midpoint, 1 perpendicular, 1 point on line, 3 other
  measures "d288" diameter of A0
  measures "d289" diameter of A1
  measures "d290" distance of L2.end L2.start
  measures "d293" angle of L5 L4
extrude "Extrusion16" [suppressed]
sketch "Sketch18" plane through (-36.1295, 16.7619, 51.6398) normal (0, 0, -1) x (-1, 0, 0)
  line L0 (65.79, 39.188) -> (51.814, 39.188)
  line L1 (51.814, 39.188) -> (51.814, -35.1)
  line L2 (51.814, -35.1) -> (65.79, -35.1)
  line L3 (65.79, -35.1) -> (65.79, 39.188)
  line L4 (64.79, -32.1) -> (64.79, 36.188) projected
  line L5 (62.79, 38.188) -> (39.4901, 38.188) projected
  line L6 (-53.17, -34.1) -> (62.79, -34.1) projected
  point P0 (-36.1295, -16.7619)
  point P1 (64.79, 37.188)
  point P2 (62.79, 39.188)
  point P3 (39.9335, 39.188)
  point P4 (39.4901, 38.188)
  dimension "d296" = 12.976
  dimension "d297" = 1
  dimension "d298" = 1
  dimension "d299" = 1
  constraints: 8 end point, 2 parallel, 1 horizontal, 1 perpendicular, 1 other
  measures "d296" distance between parallel lines of L1 L4
  measures "d298" distance between parallel lines of L2 L6
  measures "d299" distance between parallel lines of L3 L4
extrude "Extrusion17" cut sketch "Sketch18" against normal blind 6
sketch "Sketch19" plane through (-36.1295, 16.7619, 114.6398) normal (0, 0, -1) x (-1, 0, 0)
  line L0 (14.825, -26.1) -> (14.825, -32.1) projected
  line L1 (14.825, -32.1) -> (60.79, -32.1) projected
  arc A0 (60.79, -32.1) -> (62.79, -30.1) centre (60.79, -30.1) ccw projected
  line L2 (62.79, -30.1) -> (62.79, 34.188) projected
  arc A1 (62.79, 34.188) -> (60.79, 36.188) centre (60.79, 34.188) ccw projected
  line L3 (60.79, 36.188) -> (39.4901, 36.188) projected
  arc A2 (38.2222, 36.4691) -> (39.4901, 36.188) centre (39.4901, 39.188) ccw projected
  line L4 (38.2222, 36.4691) -> (26.4278, 41.9689) projected
  arc A3 (26.4278, 41.9689) -> (25.1599, 42.25) centre (25.1599, 39.25) ccw projected
  line L5 (25.1599, 42.25) -> (-23.5099, 42.25) projected
  arc A4 (-23.5099, 42.25) -> (-24.7778, 41.9689) centre (-23.5099, 39.25) ccw projected
  line L6 (-24.7778, 41.9689) -> (-36.5722, 36.4691) projected
  arc A5 (-37.8401, 36.188) -> (-36.5722, 36.4691) centre (-37.8401, 39.188) ccw projected
  line L7 (-37.8401, 36.188) -> (-51.17, 36.188) projected
  arc A6 (-51.17, 36.188) -> (-53.17, 34.188) centre (-51.17, 34.188) ccw projected
  line L8 (-53.17, 34.188) -> (-53.17, -30.1) projected
  arc A7 (-53.17, -30.1) -> (-51.17, -32.1) centre (-51.17, -30.1) ccw projected
  line L9 (-51.17, -32.1) -> (-15.375, -32.1) projected
  line L10 (-15.375, -32.1) -> (-15.375, -26.1) projected
  line L11 (-15.375, -26.1) -> (-28.95, -26.1) projected
  line L12 (-28.95, -26.1) -> (-28.95, 31.25) projected
  line L13 (-28.95, 31.25) -> (28.4, 31.25) projected
  line L14 (28.4, 31.25) -> (28.4, -26.1) projected
  line L15 (28.4, -26.1) -> (14.825, -26.1) projected
  circle A8 centre (-34.95, 27.44) radius 1.5 projected
  circle A9 centre (34.95, 27.44) radius 1.5 projected
  circle A10 centre (34.95, -22.29) radius 1.5 projected
  circle A11 centre (-34.95, -22.29) radius 1.5 projected
  circle A12 centre (-34.95, 27.44) radius 4
  circle A13 centre (-34.95, -22.29) radius 1.5 projected
  circle A14 centre (-34.95, -22.29) radius 4
  circle A15 centre (34.95, -22.29) radius 4
  circle A16 centre (34.95, 27.44) radius 1.5 projected
  circle A17 centre (34.95, 27.44) radius 4
  point P0 (-36.1295, -16.7619)
  dimension "d313" = 8
  dimension "d314" = 8
  dimension "d315" = 8
  dimension "d316" = 8
  constraints: 4 centre point, 4 coincident
  measures "d313" diameter of A12
  measures "d314" diameter of A14
  measures "d315" diameter of A15
  measures "d316" diameter of A17
extrude "Extrusion18" add sketch "Sketch19" along normal blind 3 contours A12 | A14 | A15 | A17
lip "Lip2" kind groove height 1 width 1 edges at (-92.4315, 52.9499, 57.6398) (-98.3337, 52.3642, 57.6398) (-98.9195, 18.8059, 57.6398) (-98.3337, -14.7523, 57.6398) (-92.4315, -15.3381, 57.6398) guide face at (-100.2528, 8.0913, 57.6398)
equation "\"Wall_Thickness\" = 2"
body "Solid2"
